Walllight Mount (Autodesk Fusion 360 design; units mm, degrees)
Autodesk Fusion 360 part; units mm, degrees
note: some values were not read from the file. Set by a fixed rule: which sketch regions a step uses.
sketch "Sketch1" plane through (0, 0, 0) normal (1, 0, 0) x (0, 0, -1)
  line L0 (0, 0) -> (-2, 0)
  line L1 (-2, 0) -> (-2, 14.4)
  line L2 (-2, 14.4) -> (0, 14.4)
  line L3 (0, 14.4) -> (0, 0)
  line L4 (-2, 10.9) -> (-3.8, 10.9)
  line L5 (-3.8, 10.9) -> (-3.8, 7.9)
  line L6 (-3.8, 7.9) -> (-2, 7.9)
  line L7 (-2, 7.9) -> (-2, 10.9)
  line L8 (-12.3, 13.4) -> (-3.8, 13.4)
  line L9 (-3.8, 13.4) -> (-3.8, 7.9)
  line L10 (-3.8, 7.9) -> (-12.3, 7.9)
  line L11 (-12.3, 7.9) -> (-12.3, 13.4)
  dimension "d1" = 14.4
  dimension "d2" = 2
  dimension "d3" = 1.8
  dimension "d4" = 3
  dimension "d5" = 3.5
  dimension "d6" = 8.5
  dimension "d8" = 2.5
  constraint horizontal L0
  constraint vertical L1
  constraint horizontal L2
  constraint vertical L3
  constraint coincident L0.start L3.end
  constraint horizontal L4
  constraint vertical L5
  constraint horizontal L6
  constraint vertical L7
  constraint coincident L1 L4.start
  constraint horizontal L8
  constraint vertical L9
  constraint horizontal L10
  constraint vertical L11
  constraint collinear L5 L9
  constraint coincident L5.end L6.start
  measures "d1" distance of L0.start L2.end
  measures "d2" distance of L0.start L0.end
  measures "d3" distance of L4.start L4.end
  measures "d4" distance of L4.start L6.end
  measures "d5" distance of L1.end L4.start
  measures "d6" distance of L8.start L8.end
  measures "d8" distance of L4.end L8.end
extrude "Extrude1" add sketch "Sketch1" along normal blind 30
chamfer "Chamfer1" distance 4.5 distance2 8.5 1 edges at (15, 7.9, 12.3) measured on face at (10, 9.7333, 12.3)
ref_plane "WorkPlane1" through (15, 12.15, 13.8) normal (0, 0, -1) x (0, 1, 0)
fillet "Fillet2" radius 3.5 1 edges at (15, 12.4, 12.3)
sketch "Sketch2" plane through (0, 0, 0) normal (0, 0, 1) x (1, 0, 0)
  line L0 (0, 0) -> (30, 0)
  line L1 (30, 0) -> (30, 7.9)
  line L2 (30, 7.9) -> (0, 7.9)
  line L3 (0, 7.9) -> (0, 0)
  circle A0 centre (7, 6.65) radius 2.05
  circle A1 centre (23, 6.65) radius 2.05
  circle A2 centre (23, 6.65) radius 4
  circle A3 centre (7, 6.65) radius 4
  dimension "d17" = 30
  dimension "d18" = 7.9
  dimension "d19" = 4.1
  dimension "d21" = 4.1
  dimension "d22" = 7
  dimension "d23" = 1.25
  dimension "d25" = 1.25
  dimension "d28" = 7
  dimension "d29" = 8
  dimension "d30" = 8
  constraint horizontal L0
  constraint vertical L1
  constraint horizontal L2
  constraint vertical L3
  constraint coincident L0.start L3.end
  constraint concentric A1 A2
  constraint concentric A0 A3
  measures "d17" distance of L0.start L0.end
  measures "d18" distance of L0.start L2.end
  measures "d19" diameter of A0
  measures "d21" diameter of A1
  measures "d22" distance of L1 A1.centre
  measures "d23" vertical distance of L1.end A1.centre
  measures "d25" vertical distance of L2.end A0.centre
  measures "d28" distance of L3 A0.centre
  measures "d29" diameter of A2
  measures "d30" diameter of A3
extrude "Extrude2" cut sketch "Sketch2" along normal blind 16 contours L2 A0 | L2 A0 | L2 A1 | L2 A1
extrude "Extrude3" cut sketch "Sketch2" along normal blind 16 from surface at 2 contours L2 A0 A3 | L2 A0 A3 | L2 A1 A2 | L2 A1 A2
